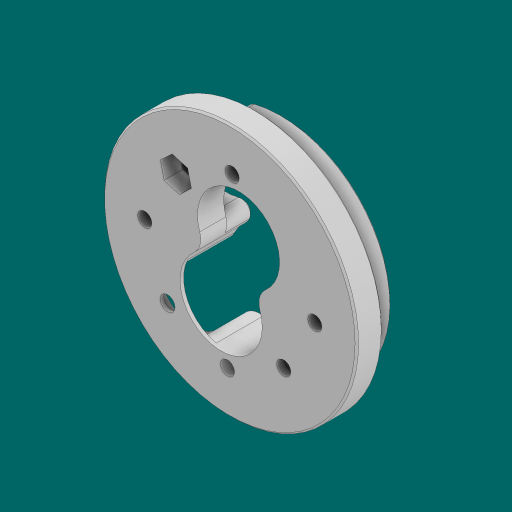
# Autodesk Inventor part: UpperRingSeat
Saved by Autodesk Inventor 2023.1 (Build 271208000, 208)
## iProperties
Created: 2022-10-30
Part Number: UpperRingSeat
Material: Generic
Document SubType Name: Modeling
Designer: zac-h
Density: 1 g/cm^3
Appearance: Default
Author: zac-h
## iProperties of the stored document UpperRingSeat_3DPrint.ipt
Created: 2022-10-31
Part Number: UpperRingSeat_3DPrint
Material: Generic
Document SubType Name: Modeling
Designer: zac-h
Density: 1 g/cm^3
Appearance: Default
Author: zac-h
Autodesk Inventor part; units mm, degrees
ref_plane "YZ Plane" through (0, 0, 0) normal (1, 0, 0) x (0, 1, 0)
ref_plane "XZ Plane" through (0, 0, 0) normal (0, 1, 0) x (-1, 0, 0)
ref_plane "XY Plane" through (0, 0, 0) normal (0, 0, 1) x (1, 0, 0)
sketch "Sketch1" plane through (0, 0, 0) normal (0, 0, 1) x (1, 0, 0)
  line L0 (15.1542, -20.8123) -> (13.6663, -19.2405) projected
  line L1 (13.6663, -19.2405) -> (15.2381, -17.7527) projected
  arc A0 (16.8906, -16.1885) -> (15.2381, -17.7527) centre (18.3343, -19.3686) ccw projected
  line L2 (16.8906, -16.1885) -> (18.4624, -14.7006) projected
  line L3 (18.4624, -14.7006) -> (19.9502, -16.2724) projected
  arc A1 (21.5144, -17.9248) -> (19.9502, -16.2724) centre (18.3343, -19.3686) ccw projected
  line L4 (21.5144, -17.9248) -> (23.0023, -19.4966) projected
  line L5 (23.0023, -19.4966) -> (21.4305, -20.9845) projected
  arc A2 (19.778, -22.5487) -> (21.4305, -20.9845) centre (18.3343, -19.3686) ccw projected
  line L6 (19.778, -22.5487) -> (18.2063, -24.0366) projected
  line L7 (18.2063, -24.0366) -> (16.7184, -22.4648) projected
  arc A3 (15.1542, -20.8123) -> (16.7184, -22.4648) centre (18.3343, -19.3686) ccw projected
  line L8 (-22.5974, -16.844) -> (-21.0256, -15.3561) projected
  line L9 (-21.0256, -15.3561) -> (-19.5378, -16.9279) projected
  arc A4 (-17.9736, -18.5804) -> (-19.5378, -16.9279) centre (-21.1537, -20.0241) ccw projected
  line L10 (-17.9736, -18.5804) -> (-16.4857, -20.1521) projected
  line L11 (-16.4857, -20.1521) -> (-18.0575, -21.64) projected
  arc A5 (-19.71, -23.2042) -> (-18.0575, -21.64) centre (-21.1537, -20.0241) ccw projected
  line L12 (-19.71, -23.2042) -> (-21.2817, -24.6921) projected
  line L13 (-21.2817, -24.6921) -> (-22.7696, -23.1203) projected
  arc A6 (-24.3338, -21.4678) -> (-22.7696, -23.1203) centre (-21.1537, -20.0241) ccw projected
  line L14 (-24.3338, -21.4678) -> (-25.8217, -19.896) projected
  line L15 (-25.8217, -19.896) -> (-24.2499, -18.4082) projected
  arc A7 (-22.5974, -16.844) -> (-24.2499, -18.4082) centre (-21.1537, -20.0241) ccw projected
  circle A8 centre (28.9141, -0.7932) radius 1.9844 projected
  circle A9 centre (-0.7932, -28.9141) radius 1.9844 projected
  circle A10 centre (-28.9141, 0.7932) radius 1.9844 projected
  circle A11 centre (0.7932, 28.9141) radius 1.9844 projected
  circle A12 centre (0, 0) radius 42.58 projected
  circle A13 centre (2.9551, 11.0414) radius 13.97
  circle A14 centre (-2.9551, -11.0414) radius 13.97
  circle A15 centre (-21.1537, -20.0241) radius 11.43
  circle A16 centre (-18.3343, 19.3686) radius 13.97
  circle A17 centre (0, 0) radius 37.465 construction
  circle A18 centre (0, 0) radius 37.215
  circle A19 centre (0.7932, 28.9141) radius 2.413
  circle A20 centre (28.9141, -0.7932) radius 2.413
  circle A21 centre (-0.7932, -28.9141) radius 2.413
  circle A22 centre (-28.9141, 0.7932) radius 2.413
  circle A23 centre (-2.9551, -11.0414) radius 2.413 projected
  circle A24 centre (2.9551, 11.0414) radius 2.413 projected
  circle A25 centre (-18.3343, 19.3686) radius 2.413 projected
  point P0 (0, 0)
  point P1 (-19.9842, -31.3941)
  point P2 (-10.1261, -23.0304)
  point P3 (-32.2786, 18.5215)
  point P4 (-32.4425, -18.233)
  point P5 (-16.8332, -9.4421)
  point P6 (-7.7591, 2.0766)
  point P7 (-10.6155, 7.7247)
  point P8 (-16.7241, 33.2455)
  point P9 (-4.7638, 22.6853)
  point P10 (7.7591, -2.0766)
  dimension "d0" = 27.94
  dimension "d1" = 22.86
  dimension "d2" = 0.25
  dimension "d3" = 74.93
  dimension "d11" = 4.826
  constraints: 10 centre point, 8 coincident, 5 equal radius, 1 concentric
  measures "d0" diameter of A13
  measures "d1" diameter of A15
  measures "d2" radial gap between concentric circles of A17 A18
  measures "d3" diameter of A17
  measures "d11" diameter of A19
extrude "Extrusion1" add sketch "Sketch1" along normal blind 8.89 contours A13 A16 A18 A15 A14 | A13 A14 A15 A18 A16
sketch "Sketch2" plane through (0, 0, 8.89) normal (0, 0, 1) x (1, 0, 0)
  circle A0 centre (0, 0) radius 43.18
  circle A1 centre (0.7932, 28.9141) radius 2.413
  circle A2 centre (28.9141, -0.7932) radius 2.413
  circle A3 centre (-0.7932, -28.9141) radius 2.413
  circle A4 centre (-28.9141, 0.7932) radius 2.413
  arc A5 (7.7591, -2.0766) -> (-4.7638, 22.6853) centre (2.9551, 11.0414) ccw projected
  arc A6 (-10.1261, -23.0304) -> (7.7591, -2.0766) centre (-2.9551, -11.0414) ccw projected
  circle A7 centre (2.9551, 11.0414) radius 13.97
  circle A8 centre (-2.9551, -11.0414) radius 13.97
  arc A9 (32.2443, -18.0753) -> (10.6155, -7.7247) centre (18.3343, -19.3686) ccw projected
  circle A10 centre (18.3343, -19.3686) radius 13.97
  line L0 (0, 0) -> (-15.6399, 16.5222) construction
  circle A11 centre (-28.9141, 0.7932) radius 2.413 projected
  circle A12 centre (0.7932, 28.9141) radius 2.413 projected
  circle A13 centre (28.9141, -0.7932) radius 2.413 projected
  circle A14 centre (-0.7932, -28.9141) radius 2.413 projected
  arc A15 (-32.4425, -18.233) -> (-19.9842, -31.3941) centre (-21.1537, -20.0241) ccw projected
  circle A16 centre (-21.1537, -20.0241) radius 11.43
  arc A17 (-4.7638, 22.6853) -> (-16.7241, 33.2455) centre (-18.3343, 19.3686) ccw projected
  arc A18 (7.7591, -2.0766) -> (-4.7638, 22.6853) centre (2.9551, 11.0414) ccw projected
  arc A19 (-10.1261, -23.0304) -> (7.7591, -2.0766) centre (-2.9551, -11.0414) ccw projected
  arc A20 (-19.9842, -31.3941) -> (-10.1261, -23.0304) centre (-21.1537, -20.0241) ccw projected
  arc A21 (-19.9842, -31.3941) -> (-16.7241, 33.2455) centre (0, 0) ccw projected
  circle A22 centre (-0.7932, -28.9141) radius 2.413 projected
  circle A23 centre (28.9141, -0.7932) radius 2.413 projected
  circle A24 centre (0.7932, 28.9141) radius 2.413 projected
  line L1 (19.778, -22.5487) -> (18.2063, -24.0366) projected
  line L2 (18.2063, -24.0366) -> (16.7184, -22.4648) projected
  arc A25 (15.1542, -20.8123) -> (16.7184, -22.4648) centre (18.3343, -19.3686) ccw projected
  line L3 (15.1542, -20.8123) -> (13.6663, -19.2405) projected
  line L4 (13.6663, -19.2405) -> (15.2381, -17.7527) projected
  arc A26 (16.8906, -16.1885) -> (15.2381, -17.7527) centre (18.3343, -19.3686) ccw projected
  line L5 (16.8906, -16.1885) -> (18.4624, -14.7006) projected
  line L6 (18.4624, -14.7006) -> (19.9502, -16.2724) projected
  arc A27 (21.5144, -17.9248) -> (19.9502, -16.2724) centre (18.3343, -19.3686) ccw projected
  line L7 (21.5144, -17.9248) -> (23.0023, -19.4966) projected
  line L8 (23.0023, -19.4966) -> (21.4305, -20.9845) projected
  arc A28 (19.778, -22.5487) -> (21.4305, -20.9845) centre (18.3343, -19.3686) ccw projected
  line L9 (-17.0572, 14.0197) -> (-22.328, 15.5881)
  line L10 (-22.328, 15.5881) -> (-23.6052, 20.937)
  line L11 (-23.6052, 20.937) -> (-19.6114, 24.7175)
  line L12 (-19.6114, 24.7175) -> (-14.3406, 23.1491)
  line L13 (-14.3406, 23.1491) -> (-13.0635, 17.8001)
  line L14 (-13.0635, 17.8001) -> (-17.0572, 14.0197)
  point P0 (4.7638, -22.6853)
  point P1 (-7.7591, 2.0766)
  point P2 (-4.7638, 22.6853)
  point P3 (-16.8332, -9.4421)
  point P4 (-10.1261, -23.0304)
  point P5 (-32.4425, -18.233)
  point P6 (7.7591, -2.0766)
  point P7 (7.7591, -2.0766)
  point P8 (4.7638, -22.6853)
  point P9 (-10.1261, -23.0304)
  point P10 (7.7591, -2.0766)
  point P11 (-15.0603, 15.9099)
  dimension "d6" = 86.36
  dimension "d22" = 9.525
  constraints: 14 end point, 10 coincident, 7 centre point, 4 concentric, 2 point on circle, 1 midpoint, 1 perpendicular, 1 point on line, 19 other
  measures "d6" diameter of A0
  measures "d22" distance between parallel lines of L11 L14
extrude "Extrusion2" add sketch "Sketch2" along normal blind 8.89 contours A0 | A5 A17 A21 A10 A9 A6 | A9 A10 A21 A6 | A10 A21 A16 A6 | A10 A21
chamfer "Chamfer1" distance 0.6 angle 45 2 edges at (-43.18, 0, 8.89) (-43.18, 0, 17.78)
fillet "Fillet1" radius 6.35 4 edges at (7.7591, -2.0766, 8.89) (-10.1261, -23.0304, 8.89) (-16.8332, -9.4421, 8.89) (-7.7591, 2.0766, 8.89)
sketch "Sketch3" plane through (0, 0, 17.78) normal (0, 0, 1) x (1, 0, 0)
  arc A0 (-12.0811, -0.4643) -> (-10.2342, 6.4366) centre (-16.2293, 4.3435) ccw projected
  arc A1 (12.0811, 0.4643) -> (-10.2342, 6.4366) centre (2.9551, 11.0414) ccw projected
  arc A2 (12.0811, 0.4643) -> (10.2342, -6.4366) centre (16.2293, -4.3435) ccw projected
  arc A3 (-5.8133, -24.7159) -> (10.2342, -6.4366) centre (-2.9551, -11.0414) ccw projected
  arc A4 (-5.8133, -24.7159) -> (-12.1272, -27.036) centre (-7.1125, -30.9316) ccw projected
  arc A5 (-21.2299, -8.5944) -> (-12.1272, -27.036) centre (-21.1537, -20.0241) ccw projected
  arc A6 (-21.2299, -8.5944) -> (-15.5481, -4.9935) centre (-21.2722, -2.2445) ccw projected
  arc A7 (-12.0811, -0.4643) -> (-15.5481, -4.9935) centre (-2.9551, -11.0414) ccw projected
  line L0 (21.5144, -17.9248) -> (23.0023, -19.4966) projected
  line L1 (23.0023, -19.4966) -> (21.4305, -20.9845) projected
  arc A8 (19.778, -22.5487) -> (21.4305, -20.9845) centre (18.3343, -19.3686) ccw projected
  line L2 (19.778, -22.5487) -> (18.2063, -24.0366) projected
  line L3 (18.2063, -24.0366) -> (16.7184, -22.4648) projected
  arc A9 (15.1542, -20.8123) -> (16.7184, -22.4648) centre (18.3343, -19.3686) ccw projected
  line L4 (15.1542, -20.8123) -> (13.6663, -19.2405) projected
  line L5 (13.6663, -19.2405) -> (15.2381, -17.7527) projected
  arc A10 (16.8906, -16.1885) -> (15.2381, -17.7527) centre (18.3343, -19.3686) ccw projected
  line L6 (16.8906, -16.1885) -> (18.4624, -14.7006) projected
  line L7 (18.4624, -14.7006) -> (19.9502, -16.2724) projected
  arc A11 (21.5144, -17.9248) -> (19.9502, -16.2724) centre (18.3343, -19.3686) ccw projected
  circle A12 centre (-28.9141, 0.7932) radius 2.413 projected
  circle A13 centre (28.9141, -0.7932) radius 2.413 projected
  circle A14 centre (0.7932, 28.9141) radius 2.413 projected
  circle A15 centre (-0.7932, -28.9141) radius 2.413 projected
  circle A16 centre (0, 0) radius 42.58 projected
  circle A17 centre (18.3343, -19.3686) radius 2.413
  dimension "d16" = 4.826
  constraints: 1 centre point, 1 coincident
  measures "d16" diameter of A17
extrude "Extrusion3" add sketch "Sketch3" against normal blind 2.54 contours L0 L1 A8 L2 L3 A9 L4 L5 A10 L6 L7 A11
sketch "Sketch4" plane through (0, 0, 0) normal (0, 0, -1) x (-1, 0, 0)
  line L0 (-13.6809, -19.2559) -> (-13.6663, -19.2405) projected
  line L1 (-18.2063, -24.0366) -> (-18.1917, -24.0211) projected
  line L2 (-18.2152, -24.0281) -> (-18.2063, -24.0366) projected
  line L3 (-23.0023, -19.4966) -> (-22.9934, -19.5051) projected
  line L4 (-22.9877, -19.4812) -> (-23.0023, -19.4966) projected
  line L5 (-18.4624, -14.7006) -> (-18.477, -14.716) projected
  line L6 (-18.4535, -14.709) -> (-18.4624, -14.7006) projected
  line L7 (-13.6663, -19.2405) -> (-13.6752, -19.2321) projected
  arc A0 (19.5378, -16.9279) -> (17.9736, -18.5804) centre (21.1537, -20.0241) ccw projected
  line L8 (21.0256, -15.3561) -> (19.5378, -16.9279) projected
  line L9 (22.5974, -16.844) -> (21.0256, -15.3561) projected
  arc A1 (24.2499, -18.4082) -> (22.5974, -16.844) centre (21.1537, -20.0241) ccw projected
  line L10 (25.8217, -19.896) -> (24.2499, -18.4082) projected
  line L11 (24.3338, -21.4678) -> (25.8217, -19.896) projected
  arc A2 (22.7696, -23.1203) -> (24.3338, -21.4678) centre (21.1537, -20.0241) ccw projected
  line L12 (21.2817, -24.6921) -> (22.7696, -23.1203) projected
  line L13 (19.71, -23.2042) -> (21.2817, -24.6921) projected
  arc A3 (18.0575, -21.64) -> (19.71, -23.2042) centre (21.1537, -20.0241) ccw projected
  line L14 (16.4857, -20.1521) -> (18.0575, -21.64) projected
  line L15 (17.9736, -18.5804) -> (16.4857, -20.1521) projected
  arc A4 (33.6746, 9.2617) -> (34.1317, -7.4017) centre (28.9141, 0.7932) ccw projected
  arc A5 (33.6746, 9.2617) -> (7.4017, 34.1317) centre (0, 0) ccw projected
  arc A6 (-9.2617, 33.6746) -> (7.4017, 34.1317) centre (-0.7932, 28.9141) ccw projected
  arc A7 (-9.2617, 33.6746) -> (-34.1317, 7.4017) centre (0, 0) ccw projected
  arc A8 (-33.6746, -9.2617) -> (-34.1317, 7.4017) centre (-28.9141, -0.7932) ccw projected
  arc A9 (-33.6746, -9.2617) -> (-7.4017, -34.1317) centre (0, 0) ccw projected
  arc A10 (9.2617, -33.6746) -> (-7.4017, -34.1317) centre (0.7932, -28.9141) ccw projected
  arc A11 (9.2617, -33.6746) -> (34.1317, -7.4017) centre (0, 0) ccw projected
  line L16 (1.7129, 11.1695) -> (1.5953, 11.2808) projected
  line L17 (1.5109, 10.9561) -> (1.7129, 11.1695) projected
  line L18 (-2.827, 6.3734) -> (-2.5727, 6.642) projected
  line L19 (-2.9893, 6.5271) -> (-2.827, 6.3734) projected
  line L20 (13.6663, 19.2405) -> (13.6752, 19.2321) projected
  line L21 (13.6809, 19.2559) -> (13.6663, 19.2405) projected
  line L22 (18.2063, 24.0366) -> (18.1917, 24.0211) projected
  line L23 (18.2152, 24.0281) -> (18.2063, 24.0366) projected
  line L24 (23.0023, 19.4966) -> (22.9934, 19.5051) projected
  line L25 (22.9877, 19.4812) -> (23.0023, 19.4966) projected
  line L26 (18.4624, 14.7006) -> (18.477, 14.716) projected
  line L27 (18.4535, 14.709) -> (18.4624, 14.7006) projected
  line L28 (-1.7129, -11.1695) -> (-1.5953, -11.2808) projected
  line L29 (-1.5109, -10.9561) -> (-1.7129, -11.1695) projected
  line L30 (2.827, -6.3734) -> (2.5727, -6.642) projected
  line L31 (2.9893, -6.5271) -> (2.827, -6.3734) projected
  circle A12 centre (-18.3343, -19.3686) radius 4.191
  line L32 (1.5109, 10.9561) -> (0.6187, 7.523) projected
  line L33 (0.6187, 7.523) -> (-2.5727, 6.642) projected
  line L34 (-2.9893, 6.5271) -> (-4.3902, 6.1404) projected
  line L35 (-4.3902, 6.1404) -> (-8.092, 9.7869) projected
  line L36 (-8.092, 9.7869) -> (-6.7849, 14.8159) projected
  line L37 (-6.7849, 14.8159) -> (-1.7761, 16.1985) projected
  line L38 (-1.7761, 16.1985) -> (1.9257, 12.552) projected
  line L39 (1.9257, 12.552) -> (1.5953, 11.2808) projected
  line L40 (13.6809, 19.2559) -> (14.5607, 22.9407) projected
  line L41 (14.5607, 22.9407) -> (18.1917, 24.0211) projected
  line L42 (18.2152, 24.0281) -> (19.541, 24.4227) projected
  line L43 (19.541, 24.4227) -> (23.3146, 20.8506) projected
  line L44 (23.3146, 20.8506) -> (22.9934, 19.5051) projected
  line L45 (22.9877, 19.4812) -> (22.1079, 15.7965) projected
  line L46 (22.1079, 15.7965) -> (18.477, 14.716) projected
  line L47 (18.4535, 14.709) -> (17.1276, 14.3145) projected
  line L48 (17.1276, 14.3145) -> (13.354, 17.8866) projected
  line L49 (13.354, 17.8866) -> (13.6752, 19.2321) projected
  line L50 (-22.9877, -19.4812) -> (-22.1079, -15.7965) projected
  line L51 (-22.1079, -15.7965) -> (-18.477, -14.716) projected
  line L52 (-18.4535, -14.709) -> (-17.1276, -14.3145) projected
  line L53 (-17.1276, -14.3145) -> (-13.354, -17.8866) projected
  line L54 (-13.354, -17.8866) -> (-13.6752, -19.2321) projected
  line L55 (-13.6809, -19.2559) -> (-14.5607, -22.9407) projected
  line L56 (-14.5607, -22.9407) -> (-18.1917, -24.0211) projected
  line L57 (-18.2152, -24.0281) -> (-19.541, -24.4227) projected
  line L58 (-19.541, -24.4227) -> (-23.3146, -20.8506) projected
  line L59 (-23.3146, -20.8506) -> (-22.9934, -19.5051) projected
  line L60 (2.9893, -6.5271) -> (4.3902, -6.1404) projected
  line L61 (4.3902, -6.1404) -> (8.092, -9.7869) projected
  line L62 (8.092, -9.7869) -> (6.7849, -14.8159) projected
  line L63 (6.7849, -14.8159) -> (1.7761, -16.1985) projected
  line L64 (1.7761, -16.1985) -> (-1.9257, -12.552) projected
  line L65 (-1.9257, -12.552) -> (-1.5953, -11.2808) projected
  line L66 (-1.5109, -10.9561) -> (-0.6187, -7.523) projected
  line L67 (-0.6187, -7.523) -> (2.5727, -6.642) projected
  point P0 (0, 0)
  dimension "d19" = 8.382
  constraints: 1 centre point
  measures "d19" diameter of A12
extrude "Extrusion4" cut sketch "Sketch4" against normal up to surface (15.24 mm away) contours A12
sketch "Sketch5" plane through (0, 0, 8.89) normal (0, 0, -1) x (-1, 0, 0)
  line L0 (17.0572, 14.0197) -> (22.328, 15.5881) projected
  line L1 (13.0635, 17.8001) -> (17.0572, 14.0197) projected
  line L2 (14.3406, 23.1491) -> (13.0635, 17.8001) projected
  line L3 (19.6114, 24.7175) -> (14.3406, 23.1491) projected
  line L4 (23.6052, 20.937) -> (19.6114, 24.7175) projected
  line L5 (22.328, 15.5881) -> (23.6052, 20.937) projected
  arc A0 (32.4425, -18.233) -> (32.2786, 18.5215) centre (0, 0) ccw projected
  arc A1 (19.9842, -31.3941) -> (32.4425, -18.233) centre (21.1537, -20.0241) ccw projected
  arc A2 (16.7241, 33.2455) -> (19.9842, -31.3941) centre (0, 0) ccw projected
  arc A3 (16.7241, 33.2455) -> (4.7638, 22.6853) centre (18.3343, 19.3686) ccw projected
  arc A4 (10.6155, 7.7247) -> (4.7638, 22.6853) centre (-2.9551, 11.0414) ccw projected
  arc A5 (10.6155, 7.7247) -> (32.2786, 18.5215) centre (18.3343, 19.3686) ccw projected
  circle A6 centre (0, 0) radius 42.58 projected
  circle A7 centre (18.3343, 19.3686) radius 2.413
  dimension "d23" = 4.826
  constraints: 1 centre point, 1 coincident
  measures "d23" diameter of A7
extrude "Extrusion5" add sketch "Sketch5" against normal blind 2.54 contours L1 L2 L3 L4 L5 L0
sketch "Sketch6" plane through (0, 0, 17.78) normal (0, 0, 1) x (1, 0, 0)
  arc A0 (-12.0811, -0.4643) -> (-15.5481, -4.9935) centre (-2.9551, -11.0414) ccw projected
  circle A1 centre (-2.9551, -11.0414) radius 13.97
  circle A2 centre (18.3343, -19.3686) radius 2.413 projected
  arc A3 (-12.0811, -0.4643) -> (-10.2342, 6.4366) centre (-16.2293, 4.3435) ccw projected
  arc A4 (12.0811, 0.4643) -> (-10.2342, 6.4366) centre (2.9551, 11.0414) ccw projected
  arc A5 (12.0811, 0.4643) -> (10.2342, -6.4366) centre (16.2293, -4.3435) ccw projected
  arc A6 (-5.8133, -24.7159) -> (10.2342, -6.4366) centre (-2.9551, -11.0414) ccw projected
  arc A7 (-5.8133, -24.7159) -> (-12.1272, -27.036) centre (-7.1125, -30.9316) ccw projected
  arc A8 (-21.2299, -8.5944) -> (-12.1272, -27.036) centre (-21.1537, -20.0241) ccw projected
  arc A9 (-21.2299, -8.5944) -> (-15.5481, -4.9935) centre (-21.2722, -2.2445) ccw projected
  arc A10 (-12.0811, -0.4643) -> (-15.5481, -4.9935) centre (-2.9551, -11.0414) ccw projected
  circle A11 centre (-28.9141, 0.7932) radius 2.413 projected
  line L0 (-17.0572, 14.0197) -> (-22.328, 15.5881) projected
  line L1 (-22.328, 15.5881) -> (-23.6052, 20.937) projected
  line L2 (-23.6052, 20.937) -> (-19.6114, 24.7175) projected
  line L3 (-19.6114, 24.7175) -> (-14.3406, 23.1491) projected
  line L4 (-14.3406, 23.1491) -> (-13.0635, 17.8001) projected
  line L5 (-13.0635, 17.8001) -> (-17.0572, 14.0197) projected
  circle A12 centre (28.9141, -0.7932) radius 2.413 projected
  circle A13 centre (0.7932, 28.9141) radius 2.413 projected
  circle A14 centre (-0.7932, -28.9141) radius 2.413 projected
  circle A15 centre (0, 0) radius 42.58 projected
  circle A16 centre (-21.1537, -20.0241) radius 2.54
  point P0 (-5.8133, -24.7159)
  point P1 (-15.5481, -4.9935)
  dimension "d29" = 5.08
  constraints: 2 coincident, 1 centre point, 3 other
  measures "d29" diameter of A16
extrude "Extrusion6" add sketch "Sketch6" against normal blind 1.2 contours A1 A7 A8 A9
fillet "Fillet2" radius 3.175 6 edges at (-19.9842, -31.3941, 4.445) (-32.4425, -18.233, 4.445) (-10.6155, 7.7247, 4.445) (-32.2786, 18.5215, 4.445) (-16.7241, 33.2455, 4.445) (-4.7638, 22.6853, 4.445)
chamfer "Chamfer2" distance 0.6 angle 45 19 edges at (37.1314, -2.4933, 0) (-11.1476, 33.7172, 0) (-7.6262, 28.3406, 0) (-4.1911, 24.1493, 0) (14.9774, 18.1564, 0) (10.0952, -2.7018, 0) (7.5433, -20.258, 0) (-9.3027, -24.9712, 0) (-13.1392, -28.1735, 0) (-15.5336, -32.1352, 0) (-23.045, 6.2168, 0) (-33.0554, 12.9793, 0) (-37.2122, -0.4539, 0) (-32.9385, -13.7485, 0) (-26.0163, -9.68, 0) (-17.873, -7.6081, 0) (-14.0482, -2.5501, 0) (-11.2088, 0.4556, 0) (-10.9575, 5.0176, 0)
body "Solid1"
